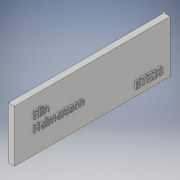
# Autodesk Inventor part: Namnbrica
Saved by Autodesk Inventor 2018 (Build 220112000, 112)
## iProperties
Created: 2018-08-23
Part Number: Namnbrica
Material: Generic
Document SubType Name: Modeling
Designer: annhed2
Density: 1 g/cm^3
Appearance: Default
Author: annhed2
Autodesk Inventor part; units mm, degrees
ref_plane "YZ Plane" through (0, 0, 0) normal (1, 0, 0) x (0, 1, 0)
ref_plane "XZ Plane" through (0, 0, 0) normal (0, 1, 0) x (-1, 0, 0)
ref_plane "XY Plane" through (0, 0, 0) normal (0, 0, 1) x (1, 0, 0)
sketch "Sketch1" plane through (0, 0, 0) normal (1, 0, 0) x (0, 1, 0)
  line L0 (0, 0) -> (-75, 0)
  line L1 (-75, 0) -> (-75, -25)
  line L2 (-75, -25) -> (0, -25)
  line L3 (0, -25) -> (0, 0)
  dimension "d0" = 75
  dimension "d1" = 25
  constraints: 8 end point, 2 parallel, 1 horizontal, 1 perpendicular
  measures "d0" distance of L2.end L1.end
  measures "d1" distance of L1.end L0.end
extrude "Extrusion1" add sketch "Sketch1" along normal blind 3
sketch "Sketch2" plane through (3, 0, 0) normal (1, 0, 0) x (0, 0, -1)
  line L0 (6.1236, -66.3795) -> (6.1236, -53.1526) construction
  line L1 (6.1236, -53.1526) -> (54.8672, -53.1526) construction
  line L2 (54.8672, -53.1526) -> (54.8672, -66.3795) construction
  line L3 (54.8672, -66.3795) -> (6.1236, -66.3795) construction
  line L4 (9.7796, -66.0249) -> (6.2796, -66.0249)
  line L5 (6.2796, -66.0249) -> (6.2796, -63.8353)
  line L6 (6.2796, -63.8353) -> (6.6937, -63.8353)
  line L7 (6.6937, -63.8353) -> (6.6937, -65.5598)
  line L8 (6.6937, -65.5598) -> (7.6523, -65.5598)
  line L9 (7.6523, -65.5598) -> (7.6523, -63.9516)
  line L10 (7.6523, -63.9516) -> (8.0664, -63.9516)
  line L11 (8.0664, -63.9516) -> (8.0664, -65.5598)
  line L12 (8.0664, -65.5598) -> (9.3655, -65.5598)
  line L13 (9.3655, -65.5598) -> (9.3655, -63.8353)
  line L14 (9.3655, -63.8353) -> (9.7796, -63.8353)
  line L15 (9.7796, -63.8353) -> (9.7796, -66.0249)
  line L16 (9.7796, -62.9078) -> (9.7796, -63.3503)
  line L17 (9.7796, -63.3503) -> (6.1236, -63.3503)
  line L18 (6.1236, -63.3503) -> (6.1236, -62.9078)
  line L19 (6.1236, -62.9078) -> (9.7796, -62.9078)
  line L20 (9.7796, -61.8074) -> (9.7796, -62.2498)
  line L21 (9.7796, -62.2498) -> (7.1531, -62.2498)
  line L22 (7.1531, -62.2498) -> (7.1531, -61.8074)
  line L23 (7.1531, -61.8074) -> (9.7796, -61.8074)
  line L24 (6.7164, -61.7762) -> (6.7164, -62.2782)
  line L25 (6.7164, -62.2782) -> (6.2569, -62.2782)
  line L26 (6.2569, -62.2782) -> (6.2569, -61.7762)
  line L27 (6.2569, -61.7762) -> (6.7164, -61.7762)
  line L28 (9.7796, -59.0958) -> (9.7796, -59.5383)
  line L29 (9.7796, -59.5383) -> (8.282, -59.5383)
  spline S0 degree 2 poles (8.282, -59.5383) (8.1005, -59.5383) (7.7885, -59.5723) (7.6949, -59.6234) knots 0 0 0 1 2 2 2
  spline S1 degree 2 poles (7.6949, -59.6234) (7.5956, -59.6773) (7.4992, -59.8702) (7.4992, -60.0347) knots 0 0 0 1 2 2 2
  spline S2 degree 2 poles (7.4992, -60.0347) (7.4992, -60.1992) (7.675, -60.548) (7.8168, -60.7154) knots 0 0 0 1 2 2 2
  line L30 (7.8168, -60.7154) -> (9.7796, -60.7154)
  line L31 (9.7796, -60.7154) -> (9.7796, -61.1578)
  line L32 (9.7796, -61.1578) -> (7.1531, -61.1578)
  line L33 (7.1531, -61.1578) -> (7.1531, -60.7154)
  line L34 (7.1531, -60.7154) -> (7.4453, -60.7154)
  spline S3 degree 2 poles (7.4453, -60.7154) (7.2666, -60.5168) (7.0794, -60.1339) (7.0794, -59.9184) knots 0 0 0 1 2 2 2
  spline S4 degree 2 poles (7.0794, -59.9184) (7.0794, -59.5326) (7.5899, -59.0958) (8.0749, -59.0958) knots 0 0 0 1 2 2 2
  line L35 (8.0749, -59.0958) -> (9.7796, -59.0958)
  line L36 (15.5422, -63.4836) -> (15.5422, -63.9488)
  line L37 (15.5422, -63.9488) -> (13.8291, -63.9488)
  line L38 (13.8291, -63.9488) -> (13.8291, -65.5598)
  line L39 (13.8291, -65.5598) -> (15.5422, -65.5598)
  line L40 (15.5422, -65.5598) -> (15.5422, -66.0249)
  line L41 (15.5422, -66.0249) -> (12.0422, -66.0249)
  line L42 (12.0422, -66.0249) -> (12.0422, -65.5598)
  line L43 (12.0422, -65.5598) -> (13.415, -65.5598)
  line L44 (13.415, -65.5598) -> (13.415, -63.9488)
  line L45 (13.415, -63.9488) -> (12.0422, -63.9488)
  line L46 (12.0422, -63.9488) -> (12.0422, -63.4836)
  line L47 (12.0422, -63.4836) -> (15.5422, -63.4836)
  spline S5 degree 2 poles (15.6018, -61.6684) (15.6018, -62.298) (14.8955, -62.9901) (14.2432, -62.9901) knots 0 0 0 1 2 2 2
  spline S6 degree 2 poles (14.2432, -62.9901) (13.6022, -62.9901) (12.8421, -62.3179) (12.8421, -61.7762) knots 0 0 0 1 2 2 2
  spline S7 degree 2 poles (12.8421, -61.7762) (12.8421, -61.5322) (12.9839, -61.155) (13.1342, -61.016) knots 0 0 0 1 2 2 2
  spline S8 degree 2 poles (13.1342, -61.016) (13.2845, -60.8742) (13.7185, -60.7239) (14.0333, -60.7239) knots 0 0 0 1 2 2 2
  line L48 (14.0333, -60.7239) -> (14.2744, -60.7239)
  line L49 (14.2744, -60.7239) -> (14.2744, -62.542)
  spline S9 degree 2 poles (14.2744, -62.542) (14.731, -62.542) (15.216, -62.0825) (15.216, -61.6741) knots 0 0 0 1 2 2 2
  spline S10 degree 2 poles (15.216, -61.6741) (15.216, -61.5294) (15.1508, -61.2486) (15.0998, -61.1352) knots 0 0 0 1 2 2 2
  spline S11 degree 2 poles (15.0998, -61.1352) (15.043, -61.016) (14.9438, -60.8515) (14.8984, -60.7976) knots 0 0 0 1 2 2 2
  line L50 (14.8984, -60.7976) -> (14.8984, -60.7721)
  line L51 (14.8984, -60.7721) -> (15.3806, -60.7721)
  spline S12 degree 2 poles (15.3806, -60.7721) (15.4118, -60.8487) (15.5025, -61.0813) (15.528, -61.172) knots 0 0 0 1 2 2 2
  spline S13 degree 2 poles (15.528, -61.172) (15.5649, -61.2997) (15.6018, -61.5095) (15.6018, -61.6684) knots 0 0 0 1 2 2 2
  spline S14 degree 2 poles (13.9369, -61.155) (13.7582, -61.1607) (13.4972, -61.2344) (13.4093, -61.3053) knots 0 0 0 1 2 2 2
  spline S15 degree 2 poles (13.4093, -61.3053) (13.3101, -61.3819) (13.2051, -61.623) (13.2051, -61.8017) knots 0 0 0 1 2 2 2
  spline S16 degree 2 poles (13.2051, -61.8017) (13.2051, -61.9775) (13.3101, -62.2243) (13.4122, -62.3264) knots 0 0 0 1 2 2 2
  spline S17 degree 2 poles (13.4122, -62.3264) (13.5171, -62.4257) (13.7695, -62.5278) (13.9369, -62.542) knots 0 0 0 1 2 2 2
  line L52 (13.9369, -62.542) -> (13.9369, -61.155)
  line L53 (15.5422, -59.8248) -> (15.5422, -60.2672)
  line L54 (15.5422, -60.2672) -> (11.8862, -60.2672)
  line L55 (11.8862, -60.2672) -> (11.8862, -59.8248)
  line L56 (11.8862, -59.8248) -> (15.5422, -59.8248)
  line L57 (15.5422, -56.1971) -> (14.022, -56.1971)
  spline S18 degree 2 poles (14.022, -56.1971) (13.8404, -56.1971) (13.5313, -56.2255) (13.4462, -56.2709) knots 0 0 0 1 2 2 2
  spline S19 degree 2 poles (13.4462, -56.2709) (13.3526, -56.3163) (13.2618, -56.4893) (13.2618, -56.6396) knots 0 0 0 1 2 2 2
  spline S20 degree 2 poles (13.2618, -56.6396) (13.2618, -56.7758) (13.4292, -57.0877) (13.588, -57.2523) knots 0 0 0 1 2 2 2
  spline S21 degree 2 poles (13.588, -57.2523) (13.6277, -57.2494) (13.7383, -57.2437) (13.8121, -57.2437) knots 0 0 0 1 2 2 2
  line L58 (13.8121, -57.2437) -> (15.5422, -57.2437)
  line L59 (15.5422, -57.2437) -> (15.5422, -57.6862)
  line L60 (15.5422, -57.6862) -> (14.022, -57.6862)
  spline S22 degree 2 poles (14.022, -57.6862) (13.8404, -57.6862) (13.5313, -57.7146) (13.4462, -57.7599) knots 0 0 0 1 2 2 2
  spline S23 degree 2 poles (13.4462, -57.7599) (13.3526, -57.8053) (13.2618, -57.9783) (13.2618, -58.1287) knots 0 0 0 1 2 2 2
  spline S24 degree 2 poles (13.2618, -58.1287) (13.2618, -58.2705) (13.4405, -58.5853) (13.5795, -58.7328) knots 0 0 0 1 2 2 2
  line L61 (13.5795, -58.7328) -> (15.5422, -58.7328)
  line L62 (15.5422, -58.7328) -> (15.5422, -59.1753)
  line L63 (15.5422, -59.1753) -> (12.9158, -59.1753)
  line L64 (12.9158, -59.1753) -> (12.9158, -58.7328)
  line L65 (12.9158, -58.7328) -> (13.2051, -58.7328)
  spline S25 degree 2 poles (13.2051, -58.7328) (13.0321, -58.5598) (12.8421, -58.2194) (12.8421, -58.0152) knots 0 0 0 1 2 2 2
  spline S26 degree 2 poles (12.8421, -58.0152) (12.8421, -57.7826) (13.0548, -57.4224) (13.2959, -57.3288) knots 0 0 0 1 2 2 2
  spline S27 degree 2 poles (13.2959, -57.3288) (13.0718, -57.1275) (12.8421, -56.7474) (12.8421, -56.5262) knots 0 0 0 1 2 2 2
  spline S28 degree 2 poles (12.8421, -56.5262) (12.8421, -56.356) (12.947, -56.078) (13.0661, -55.9759) knots 0 0 0 1 2 2 2
  spline S29 degree 2 poles (13.0661, -55.9759) (13.1853, -55.871) (13.5426, -55.7547) (13.8121, -55.7547) knots 0 0 0 1 2 2 2
  line L66 (13.8121, -55.7547) -> (15.5422, -55.7547)
  line L67 (15.5422, -55.7547) -> (15.5422, -56.1971)
  spline S30 degree 2 poles (15.6018, -53.9933) (15.6018, -54.623) (14.8955, -55.3151) (14.2432, -55.3151) knots 0 0 0 1 2 2 2
  spline S31 degree 2 poles (14.2432, -55.3151) (13.6022, -55.3151) (12.8421, -54.6429) (12.8421, -54.1011) knots 0 0 0 1 2 2 2
  spline S32 degree 2 poles (12.8421, -54.1011) (12.8421, -53.8572) (12.9839, -53.48) (13.1342, -53.341) knots 0 0 0 1 2 2 2
  spline S33 degree 2 poles (13.1342, -53.341) (13.2845, -53.1992) (13.7185, -53.0488) (14.0333, -53.0488) knots 0 0 0 1 2 2 2
  line L68 (14.0333, -53.0488) -> (14.2744, -53.0488)
  line L69 (14.2744, -53.0488) -> (14.2744, -54.8669)
  spline S34 degree 2 poles (14.2744, -54.8669) (14.731, -54.8669) (15.216, -54.4074) (15.216, -53.999) knots 0 0 0 1 2 2 2
  spline S35 degree 2 poles (15.216, -53.999) (15.216, -53.8544) (15.1508, -53.5736) (15.0998, -53.4601) knots 0 0 0 1 2 2 2
  spline S36 degree 2 poles (15.0998, -53.4601) (15.043, -53.341) (14.9438, -53.1765) (14.8984, -53.1226) knots 0 0 0 1 2 2 2
  line L70 (14.8984, -53.1226) -> (14.8984, -53.0971)
  line L71 (14.8984, -53.0971) -> (15.3806, -53.0971)
  spline S37 degree 2 poles (15.3806, -53.0971) (15.4118, -53.1736) (15.5025, -53.4062) (15.528, -53.497) knots 0 0 0 1 2 2 2
  spline S38 degree 2 poles (15.528, -53.497) (15.5649, -53.6246) (15.6018, -53.8345) (15.6018, -53.9933) knots 0 0 0 1 2 2 2
  spline S39 degree 2 poles (13.9369, -53.48) (13.7582, -53.4856) (13.4972, -53.5594) (13.4093, -53.6303) knots 0 0 0 1 2 2 2
  spline S40 degree 2 poles (13.4093, -53.6303) (13.3101, -53.7069) (13.2051, -53.948) (13.2051, -54.1266) knots 0 0 0 1 2 2 2
  spline S41 degree 2 poles (13.2051, -54.1266) (13.2051, -54.3025) (13.3101, -54.5493) (13.4122, -54.6514) knots 0 0 0 1 2 2 2
  spline S42 degree 2 poles (13.4122, -54.6514) (13.5171, -54.7506) (13.7695, -54.8527) (13.9369, -54.8669) knots 0 0 0 1 2 2 2
  line L72 (13.9369, -54.8669) -> (13.9369, -53.48)
  line L73 (13.3895, -51.2081) -> (13.3895, -51.2308)
  spline S43 degree 2 poles (13.3895, -51.2308) (13.3753, -51.2818) (13.3696, -51.3924) (13.3696, -51.469) knots 0 0 0 1 2 2 2
  spline S44 degree 2 poles (13.3696, -51.469) (13.3696, -51.6477) (13.5256, -51.9994) (13.6788, -52.1582) knots 0 0 0 1 2 2 2
  line L74 (13.6788, -52.1582) -> (15.5422, -52.1582)
  line L75 (15.5422, -52.1582) -> (15.5422, -52.6007)
  line L76 (15.5422, -52.6007) -> (12.9158, -52.6007)
  line L77 (12.9158, -52.6007) -> (12.9158, -52.1582)
  line L78 (12.9158, -52.1582) -> (13.3072, -52.1582)
  spline S45 degree 2 poles (13.3072, -52.1582) (13.0917, -51.9172) (12.9158, -51.557) (12.9158, -51.3868) knots 0 0 0 1 2 2 2
  spline S46 degree 2 poles (12.9158, -51.3868) (12.9158, -51.3187) (12.9215, -51.2506) (12.93, -51.2081) knots 0 0 0 1 2 2 2
  line L79 (12.93, -51.2081) -> (13.3895, -51.2081)
  spline S47 degree 2 poles (15.6046, -50.1558) (15.6046, -50.4196) (15.4628, -50.8762) (15.3834, -51.0266) knots 0 0 0 1 2 2 2
  line L80 (15.3834, -51.0266) -> (14.887, -51.0266)
  line L81 (14.887, -51.0266) -> (14.887, -51.0039)
  spline S48 degree 2 poles (14.887, -51.0039) (14.9324, -50.9471) (15.0402, -50.794) (15.0998, -50.6664) knots 0 0 0 1 2 2 2
  spline S49 degree 2 poles (15.0998, -50.6664) (15.1536, -50.5557) (15.2331, -50.2835) (15.2331, -50.1388) knots 0 0 0 1 2 2 2
  spline S50 degree 2 poles (15.2331, -50.1388) (15.2331, -50.0339) (15.1848, -49.7928) (15.1451, -49.736) knots 0 0 0 1 2 2 2
  spline S51 degree 2 poles (15.1451, -49.736) (15.0912, -49.6538) (14.9693, -49.58) (14.8445, -49.58) knots 0 0 0 1 2 2 2
  spline S52 degree 2 poles (14.8445, -49.58) (14.6885, -49.58) (14.5268, -49.7502) (14.4729, -49.9686) knots 0 0 0 1 2 2 2
  spline S53 degree 2 poles (14.4729, -49.9686) (14.4531, -50.0537) (14.3964, -50.326) (14.3652, -50.4423) knots 0 0 0 1 2 2 2
  spline S54 degree 2 poles (14.3652, -50.4423) (14.2772, -50.7429) (13.9142, -51.0152) (13.6561, -51.0152) knots 0 0 0 1 2 2 2
  spline S55 degree 2 poles (13.6561, -51.0152) (13.2987, -51.0152) (12.8534, -50.4792) (12.8534, -50.0367) knots 0 0 0 1 2 2 2
  spline S56 degree 2 poles (12.8534, -50.0367) (12.8534, -49.8183) (12.9612, -49.3758) (13.0434, -49.2255) knots 0 0 0 1 2 2 2
  line L82 (13.0434, -49.2255) -> (13.5171, -49.2255)
  line L83 (13.5171, -49.2255) -> (13.5171, -49.2482)
  spline S57 degree 2 poles (13.5171, -49.2482) (13.381, -49.4184) (13.225, -49.8325) (13.225, -50.0452) knots 0 0 0 1 2 2 2
  spline S58 degree 2 poles (13.225, -50.0452) (13.225, -50.2636) (13.4093, -50.5642) (13.5937, -50.5642) knots 0 0 0 1 2 2 2
  spline S59 degree 2 poles (13.5937, -50.5642) (13.761, -50.5642) (13.9227, -50.3856) (13.9737, -50.187) knots 0 0 0 1 2 2 2
  spline S60 degree 2 poles (13.9737, -50.187) (13.9993, -50.0906) (14.0503, -49.8467) (14.0815, -49.7134) knots 0 0 0 1 2 2 2
  spline S61 degree 2 poles (14.0815, -49.7134) (14.1553, -49.4241) (14.4928, -49.1291) (14.7849, -49.1291) knots 0 0 0 1 2 2 2
  spline S62 degree 2 poles (14.7849, -49.1291) (14.9551, -49.1291) (15.2558, -49.2624) (15.3664, -49.3929) knots 0 0 0 1 2 2 2
  spline S63 degree 2 poles (15.3664, -49.3929) (15.4827, -49.5318) (15.6046, -49.8864) (15.6046, -50.1558) knots 0 0 0 1 2 2 2
  spline S64 degree 2 poles (15.6046, -48.0087) (15.6046, -48.2725) (15.4628, -48.7292) (15.3834, -48.8795) knots 0 0 0 1 2 2 2
  line L84 (15.3834, -48.8795) -> (14.887, -48.8795)
  line L85 (14.887, -48.8795) -> (14.887, -48.8568)
  spline S65 degree 2 poles (14.887, -48.8568) (14.9324, -48.8001) (15.0402, -48.6469) (15.0998, -48.5193) knots 0 0 0 1 2 2 2
  spline S66 degree 2 poles (15.0998, -48.5193) (15.1536, -48.4087) (15.2331, -48.1364) (15.2331, -47.9917) knots 0 0 0 1 2 2 2
  spline S67 degree 2 poles (15.2331, -47.9917) (15.2331, -47.8868) (15.1848, -47.6457) (15.1451, -47.589) knots 0 0 0 1 2 2 2
  spline S68 degree 2 poles (15.1451, -47.589) (15.0912, -47.5067) (14.9693, -47.433) (14.8445, -47.433) knots 0 0 0 1 2 2 2
  spline S69 degree 2 poles (14.8445, -47.433) (14.6885, -47.433) (14.5268, -47.6031) (14.4729, -47.8215) knots 0 0 0 1 2 2 2
  spline S70 degree 2 poles (14.4729, -47.8215) (14.4531, -47.9066) (14.3964, -48.1789) (14.3652, -48.2952) knots 0 0 0 1 2 2 2
  spline S71 degree 2 poles (14.3652, -48.2952) (14.2772, -48.5958) (13.9142, -48.8681) (13.6561, -48.8681) knots 0 0 0 1 2 2 2
  spline S72 degree 2 poles (13.6561, -48.8681) (13.2987, -48.8681) (12.8534, -48.3321) (12.8534, -47.8896) knots 0 0 0 1 2 2 2
  spline S73 degree 2 poles (12.8534, -47.8896) (12.8534, -47.6712) (12.9612, -47.2288) (13.0434, -47.0784) knots 0 0 0 1 2 2 2
  line L86 (13.0434, -47.0784) -> (13.5171, -47.0784)
  line L87 (13.5171, -47.0784) -> (13.5171, -47.1011)
  spline S74 degree 2 poles (13.5171, -47.1011) (13.381, -47.2713) (13.225, -47.6854) (13.225, -47.8981) knots 0 0 0 1 2 2 2
  spline S75 degree 2 poles (13.225, -47.8981) (13.225, -48.1165) (13.4093, -48.4172) (13.5937, -48.4172) knots 0 0 0 1 2 2 2
  spline S76 degree 2 poles (13.5937, -48.4172) (13.761, -48.4172) (13.9227, -48.2385) (13.9737, -48.0399) knots 0 0 0 1 2 2 2
  spline S77 degree 2 poles (13.9737, -48.0399) (13.9993, -47.9435) (14.0503, -47.6996) (14.0815, -47.5663) knots 0 0 0 1 2 2 2
  spline S78 degree 2 poles (14.0815, -47.5663) (14.1553, -47.277) (14.4928, -46.982) (14.7849, -46.982) knots 0 0 0 1 2 2 2
  spline S79 degree 2 poles (14.7849, -46.982) (14.9551, -46.982) (15.2558, -47.1153) (15.3664, -47.2458) knots 0 0 0 1 2 2 2
  spline S80 degree 2 poles (15.3664, -47.2458) (15.4827, -47.3847) (15.6046, -47.7393) (15.6046, -48.0087) knots 0 0 0 1 2 2 2
  spline S81 degree 2 poles (14.229, -44.4123) (14.8927, -44.4123) (15.616, -45.0505) (15.616, -45.5837) knots 0 0 0 1 2 2 2
  spline S82 degree 2 poles (15.616, -45.5837) (15.616, -46.1311) (14.87, -46.7579) (14.229, -46.7579) knots 0 0 0 1 2 2 2
  spline S83 degree 2 poles (14.229, -46.7579) (13.571, -46.7579) (12.8421, -46.1112) (12.8421, -45.5837) knots 0 0 0 1 2 2 2
  spline S84 degree 2 poles (12.8421, -45.5837) (12.8421, -45.0505) (13.5682, -44.4123) (14.229, -44.4123) knots 0 0 0 1 2 2 2
  spline S85 degree 2 poles (14.229, -44.8689) (13.7185, -44.8689) (13.2221, -45.2405) (13.2221, -45.5837) knots 0 0 0 1 2 2 2
  spline S86 degree 2 poles (13.2221, -45.5837) (13.2221, -45.9269) (13.7185, -46.3013) (14.229, -46.3013) knots 0 0 0 1 2 2 2
  spline S87 degree 2 poles (14.229, -46.3013) (14.7254, -46.3013) (15.2359, -45.9269) (15.2359, -45.5837) knots 0 0 0 1 2 2 2
  spline S88 degree 2 poles (15.2359, -45.5837) (15.2359, -45.2433) (14.7339, -44.8689) (14.229, -44.8689) knots 0 0 0 1 2 2 2
  line L88 (15.5422, -41.8965) -> (15.5422, -42.339)
  line L89 (15.5422, -42.339) -> (14.0447, -42.339)
  spline S89 degree 2 poles (14.0447, -42.339) (13.8631, -42.339) (13.5511, -42.373) (13.4575, -42.4241) knots 0 0 0 1 2 2 2
  spline S90 degree 2 poles (13.4575, -42.4241) (13.3583, -42.4779) (13.2618, -42.6708) (13.2618, -42.8353) knots 0 0 0 1 2 2 2
  spline S91 degree 2 poles (13.2618, -42.8353) (13.2618, -42.9998) (13.4377, -43.3487) (13.5795, -43.516) knots 0 0 0 1 2 2 2
  line L90 (13.5795, -43.516) -> (15.5422, -43.516)
  line L91 (15.5422, -43.516) -> (15.5422, -43.9585)
  line L92 (15.5422, -43.9585) -> (12.9158, -43.9585)
  line L93 (12.9158, -43.9585) -> (12.9158, -43.516)
  line L94 (12.9158, -43.516) -> (13.2079, -43.516)
  spline S92 degree 2 poles (13.2079, -43.516) (13.0293, -43.3175) (12.8421, -42.9346) (12.8421, -42.719) knots 0 0 0 1 2 2 2
  spline S93 degree 2 poles (12.8421, -42.719) (12.8421, -42.3333) (13.3526, -41.8965) (13.8376, -41.8965) knots 0 0 0 1 2 2 2
  line L95 (13.8376, -41.8965) -> (15.5422, -41.8965)
  point P0 (0, 0)
  constraints: 2 other
extrude "Extrusion2" add sketch "Sketch2" along normal blind 0.75
sketch "Sketch3" plane through (0, 0, 0) normal (-1, 0, 0) x (0, 0, 1)
  point P0 (0, 0)
sketch "Sketch4" plane through (3, 0, 0) normal (1, 0, 0) x (0, 0, -1)
  line L0 (18.1472, -17.5142) -> (18.1472, -10.3365) construction
  line L1 (18.1472, -10.3365) -> (36.57, -10.3365) construction
  line L2 (36.57, -10.3365) -> (36.57, -17.5142) construction
  line L3 (36.57, -17.5142) -> (18.1472, -17.5142) construction
  spline S0 degree 2 poles (20.6517, -14.7857) (20.9126, -14.7857) (21.3126, -14.9842) (21.443, -15.1487) knots 0 0 0 1 2 2 2
  spline S1 degree 2 poles (21.443, -15.1487) (21.5962, -15.3473) (21.7267, -15.7982) (21.7267, -16.1556) knots 0 0 0 1 2 2 2
  line L4 (21.7267, -16.1556) -> (21.7267, -17.1597)
  line L5 (21.7267, -17.1597) -> (18.2267, -17.1597)
  line L6 (18.2267, -17.1597) -> (18.2267, -16.2322)
  spline S2 degree 2 poles (18.2267, -16.2322) (18.2267, -15.8578) (18.2749, -15.4834) (18.3685, -15.3132) knots 0 0 0 1 2 2 2
  spline S3 degree 2 poles (18.3685, -15.3132) (18.4678, -15.1232) (18.7939, -14.9502) (19.0152, -14.9502) knots 0 0 0 1 2 2 2
  spline S4 degree 2 poles (19.0152, -14.9502) (19.2619, -14.9502) (19.6533, -15.2111) (19.7639, -15.4409) knots 0 0 0 1 2 2 2
  line L7 (19.7639, -15.4409) -> (19.781, -15.4409)
  spline S5 degree 2 poles (19.781, -15.4409) (19.866, -15.1289) (20.317, -14.7857) (20.6517, -14.7857) knots 0 0 0 1 2 2 2
  spline S6 degree 2 poles (20.6716, -15.2707) (20.473, -15.2707) (20.2178, -15.3841) (20.127, -15.5543) knots 0 0 0 1 2 2 2
  spline S7 degree 2 poles (20.127, -15.5543) (20.0703, -15.6649) (20.0362, -15.9259) (20.0362, -16.1669) knots 0 0 0 1 2 2 2
  line L8 (20.0362, -16.1669) -> (20.0362, -16.6945)
  line L9 (20.0362, -16.6945) -> (21.3296, -16.6945)
  line L10 (21.3296, -16.6945) -> (21.3296, -16.3173)
  spline S8 degree 2 poles (21.3296, -16.3173) (21.3296, -16.011) (21.2729, -15.6593) (21.1821, -15.5231) knots 0 0 0 1 2 2 2
  spline S9 degree 2 poles (21.1821, -15.5231) (21.0885, -15.3926) (20.8559, -15.2707) (20.6716, -15.2707) knots 0 0 0 1 2 2 2
  spline S10 degree 2 poles (19.0804, -15.4352) (18.9556, -15.4352) (18.7684, -15.5203) (18.7145, -15.6139) knots 0 0 0 1 2 2 2
  spline S11 degree 2 poles (18.7145, -15.6139) (18.6521, -15.7273) (18.6237, -16.0024) (18.6237, -16.2492) knots 0 0 0 1 2 2 2
  line L11 (18.6237, -16.2492) -> (18.6237, -16.6945)
  line L12 (18.6237, -16.6945) -> (19.6477, -16.6945)
  line L13 (19.6477, -16.6945) -> (19.6477, -16.1669)
  spline S12 degree 2 poles (19.6477, -16.1669) (19.6477, -15.9486) (19.6023, -15.7415) (19.5314, -15.6309) knots 0 0 0 1 2 2 2
  spline S13 degree 2 poles (19.5314, -15.6309) (19.4633, -15.5231) (19.2449, -15.4352) (19.0804, -15.4352) knots 0 0 0 1 2 2 2
  line L14 (21.7267, -13.5065) -> (18.6408, -13.5065)
  line L15 (18.6408, -13.5065) -> (18.6408, -14.6807)
  line L16 (18.6408, -14.6807) -> (18.2267, -14.6807)
  line L17 (18.2267, -14.6807) -> (18.2267, -11.8671)
  line L18 (18.2267, -11.8671) -> (18.6408, -11.8671)
  line L19 (18.6408, -11.8671) -> (18.6408, -13.0413)
  line L20 (18.6408, -13.0413) -> (21.7267, -13.0413)
  line L21 (21.7267, -13.0413) -> (21.7267, -13.5065)
  line L22 (21.7267, -11.5126) -> (18.2267, -11.5126)
  line L23 (18.2267, -11.5126) -> (18.2267, -9.3229)
  line L24 (18.2267, -9.3229) -> (18.6408, -9.3229)
  line L25 (18.6408, -9.3229) -> (18.6408, -11.0474)
  line L26 (18.6408, -11.0474) -> (19.5994, -11.0474)
  line L27 (19.5994, -11.0474) -> (19.5994, -9.4392)
  line L28 (19.5994, -9.4392) -> (20.0135, -9.4392)
  line L29 (20.0135, -9.4392) -> (20.0135, -11.0474)
  line L30 (20.0135, -11.0474) -> (21.3126, -11.0474)
  line L31 (21.3126, -11.0474) -> (21.3126, -9.3229)
  line L32 (21.3126, -9.3229) -> (21.7267, -9.3229)
  line L33 (21.7267, -9.3229) -> (21.7267, -11.5126)
  line L34 (21.7267, -6.9291) -> (21.7267, -8.6366)
  line L35 (21.7267, -8.6366) -> (21.3693, -8.6366)
  line L36 (21.3693, -8.6366) -> (21.3693, -8.0012)
  line L37 (21.3693, -8.0012) -> (19.0237, -8.0012)
  line L38 (19.0237, -8.0012) -> (19.0237, -8.6366)
  line L39 (19.0237, -8.6366) -> (18.7032, -8.6366)
  spline S14 degree 2 poles (18.7032, -8.6366) (18.7032, -8.2763) (18.4989, -7.936) (18.2153, -7.9133) knots 0 0 0 1 2 2 2
  line L40 (18.2153, -7.9133) -> (18.2153, -7.5503)
  line L41 (18.2153, -7.5503) -> (21.3693, -7.5503)
  line L42 (21.3693, -7.5503) -> (21.3693, -6.9291)
  line L43 (21.3693, -6.9291) -> (21.7267, -6.9291)
  spline S15 degree 2 poles (21.8061, -5.2273) (21.8061, -5.4883) (21.6501, -5.9165) (21.5054, -6.0669) knots 0 0 0 1 2 2 2
  spline S16 degree 2 poles (21.5054, -6.0669) (21.3636, -6.2144) (20.9779, -6.3675) (20.7595, -6.3675) knots 0 0 0 1 2 2 2
  spline S17 degree 2 poles (20.7595, -6.3675) (20.4759, -6.3675) (19.9994, -6.064) (19.8575, -5.7747) knots 0 0 0 1 2 2 2
  line L44 (19.8575, -5.7747) -> (19.8434, -5.7747)
  spline S18 degree 2 poles (19.8434, -5.7747) (19.693, -6.0328) (19.3357, -6.2824) (19.069, -6.2824) knots 0 0 0 1 2 2 2
  spline S19 degree 2 poles (19.069, -6.2824) (18.6748, -6.2824) (18.1472, -5.6868) (18.1472, -5.2273) knots 0 0 0 1 2 2 2
  spline S20 degree 2 poles (18.1472, -5.2273) (18.1472, -4.7508) (18.6464, -4.1751) (19.0378, -4.1751) knots 0 0 0 1 2 2 2
  spline S21 degree 2 poles (19.0378, -4.1751) (19.2733, -4.1751) (19.7327, -4.4502) (19.8632, -4.7083) knots 0 0 0 1 2 2 2
  line L45 (19.8632, -4.7083) -> (19.8774, -4.7083)
  spline S22 degree 2 poles (19.8774, -4.7083) (20.0192, -4.402) (20.4276, -4.0871) (20.751, -4.0871) knots 0 0 0 1 2 2 2
  spline S23 degree 2 poles (20.751, -4.0871) (21.1991, -4.0871) (21.8061, -4.7395) (21.8061, -5.2273) knots 0 0 0 1 2 2 2
  spline S24 degree 2 poles (20.7964, -4.5693) (20.5808, -4.5693) (20.3255, -4.7395) (20.1951, -4.9806) knots 0 0 0 1 2 2 2
  spline S25 degree 2 poles (20.1951, -4.9806) (20.1497, -5.06) (20.0447, -5.3266) (19.9767, -5.4939) knots 0 0 0 1 2 2 2
  spline S26 degree 2 poles (19.9767, -5.4939) (20.1043, -5.6868) (20.4844, -5.8939) (20.7254, -5.8939) knots 0 0 0 1 2 2 2
  spline S27 degree 2 poles (20.7254, -5.8939) (21.0431, -5.8939) (21.4572, -5.511) (21.4572, -5.2216) knots 0 0 0 1 2 2 2
  spline S28 degree 2 poles (21.4572, -5.2216) (21.4572, -4.9267) (21.1027, -4.5693) (20.7964, -4.5693) knots 0 0 0 1 2 2 2
  spline S29 degree 2 poles (19.0435, -4.6345) (18.8081, -4.6345) (18.4933, -4.9494) (18.4933, -5.2302) knots 0 0 0 1 2 2 2
  spline S30 degree 2 poles (18.4933, -5.2302) (18.4933, -5.4854) (18.7741, -5.8116) (19.0152, -5.8116) knots 0 0 0 1 2 2 2
  spline S31 degree 2 poles (19.0152, -5.8116) (19.1882, -5.8116) (19.4293, -5.6443) (19.5257, -5.4769) knots 0 0 0 1 2 2 2
  spline S32 degree 2 poles (19.5257, -5.4769) (19.5654, -5.406) (19.7044, -5.1054) (19.7441, -4.9834) knots 0 0 0 1 2 2 2
  spline S33 degree 2 poles (19.7441, -4.9834) (19.5881, -4.7792) (19.2562, -4.6345) (19.0435, -4.6345) knots 0 0 0 1 2 2 2
  point P0 (0, 0)
  constraints: 2 other
extrude "Extrusion3" add sketch "Sketch4" along normal blind 0.75
sketch "Sketch5" plane through (0, 0, 0) normal (-1, 0, 0) x (0, 0, 1)
  circle A0 centre (-13.6836, -36.6653) radius 5
  point P0 (0, 0)
  dimension "d8" = 10
  constraints: 1 centre point
  measures "d8" diameter of A0
extrude "Extrusion4" cut sketch "Sketch5" against normal blind 1.5
body "Solid1"
